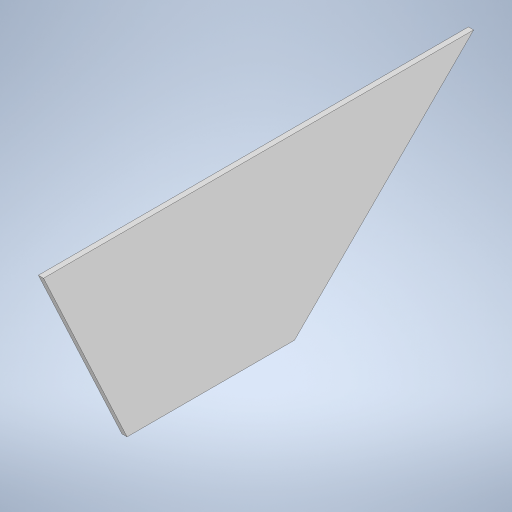
# Autodesk Inventor part: Flu-ExpansionSidesRS3
Saved by Autodesk Inventor 2024.3 (Build 283343000, 343)
## iProperties
Created: 2025-06-18
Part Number: Flu-ExpansionSidesRS3
Material: Generic
Document SubType Name: Modeling
Designer: ajclo
Density: 1 g/cm^3
Appearance: Default
Author: ajclo
Autodesk Inventor part; units mm, degrees
ref_plane "YZ Plane" through (0, 0, 0) normal (1, 0, 0) x (0, 1, 0)
ref_plane "XZ Plane" through (0, 0, 0) normal (0, 1, 0) x (-1, 0, 0)
ref_plane "XY Plane" through (0, 0, 0) normal (0, 0, 1) x (1, 0, 0)
sketch "Sketch1" plane through (0, 0, 0) normal (1, 0, 0) x (0, 1, 0)
  line L0 (0, 0) -> (103.8212, 0)
  line L1 (103.8212, 0) -> (103.8212, -97)
  line L2 (103.8212, -97) -> (0, -97)
  line L3 (0, -97) -> (0, 0)
  line L4 (0, 0) -> (103.8212, 48.4126)
  line L5 (103.8212, 48.4126) -> (103.8212, 0)
  line L6 (103.8212, -97) -> (103.8212, -200.8212)
  line L7 (103.8212, -200.8212) -> (0, -97)
  dimension "d0" = 97
  dimension "d1" = 114.554
  dimension "d2" = 45
  dimension "d3" = 25
  constraints: 16 end point, 2 parallel, 2 perpendicular, 2 point on line, 1 collinear, 1 horizontal, 1 vertical
  measures "d0" distance of L0.end L1.end
  measures "d1" distance of L0.start L4.end
  measures "d2" angle of L2 L7
  measures "d3" angle of L0 L4
extrude "Extrusion1" add sketch "Sketch1" along normal blind 3
body "Solid1"
